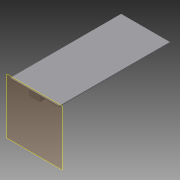
# Autodesk Inventor part: Flat Bearing
Saved by Autodesk Inventor 2014 (Build 180170000, 170)
## iProperties
Created: 2015-02-08
Part Number: Flat Bearing
Material: Generic
Document SubType Name: Modeling
Designer: Spooner
Density: 1 g/cm^3
Appearance: Default
Author: Spooner
Autodesk Inventor part; units mm, degrees
ref_plane "YZ Plane" through (0, 0, 0) normal (1, 0, 0) x (0, 1, 0)
ref_plane "XZ Plane" through (0, 0, 0) normal (0, 1, 0) x (-1, 0, 0)
ref_plane "XY Plane" through (0, 0, 0) normal (0, 0, 1) x (1, 0, 0)
ref_plane "Work Plane1" through (0, 0, 0) normal (0, 0, 1) x (1, 0, 0)
sketch "Sketch1" plane through (0, 0, 0) normal (0, 0, 1) x (1, 0, 0)
  circle A0 centre (0, 0) radius 2.413 projected
  line L0 (-4.7444, -6.5405) -> (4.7444, -6.5405) projected
  line L1 (4.7444, -6.5405) -> (10.16, -11.9561) projected
  line L2 (10.16, -11.9561) -> (10.16, -16.002) projected
  line L3 (10.16, -16.002) -> (6.985, -16.002) projected
  line L4 (6.985, -16.002) -> (6.985, -15.24) projected
  line L5 (6.985, -15.24) -> (4.445, -15.24) projected
  line L6 (4.445, -15.24) -> (4.445, -19.05) projected
  line L7 (4.445, -19.05) -> (19.05, -19.05) projected
  line L8 (19.05, -19.05) -> (19.05, -4.445) projected
  line L9 (19.05, -4.445) -> (15.24, -4.445) projected
  line L10 (15.24, -4.445) -> (15.24, -6.985) projected
  line L11 (15.24, -6.985) -> (16.002, -6.985) projected
  line L12 (16.002, -6.985) -> (16.002, -10.16) projected
  line L13 (16.002, -10.16) -> (11.9561, -10.16) projected
  line L14 (11.9561, -10.16) -> (6.5405, -4.7444) projected
  line L15 (6.5405, -4.7444) -> (6.5405, 4.7444) projected
  line L16 (6.5405, 4.7444) -> (11.9561, 10.16) projected
  line L17 (11.9561, 10.16) -> (16.002, 10.16) projected
  line L18 (16.002, 10.16) -> (16.002, 6.985) projected
  line L19 (16.002, 6.985) -> (15.24, 6.985) projected
  line L20 (15.24, 6.985) -> (15.24, 4.445) projected
  line L21 (15.24, 4.445) -> (19.05, 4.445) projected
  line L22 (19.05, 4.445) -> (19.05, 19.05) projected
  line L23 (19.05, 19.05) -> (4.445, 19.05) projected
  line L24 (4.445, 19.05) -> (4.445, 15.24) projected
  line L25 (4.445, 15.24) -> (6.985, 15.24) projected
  line L26 (6.985, 15.24) -> (6.985, 16.002) projected
  line L27 (6.985, 16.002) -> (10.16, 16.002) projected
  line L28 (10.16, 16.002) -> (10.16, 11.9561) projected
  line L29 (10.16, 11.9561) -> (4.7444, 6.5405) projected
  line L30 (4.7444, 6.5405) -> (-4.7444, 6.5405) projected
  line L31 (-4.7444, 6.5405) -> (-10.16, 11.9561) projected
  line L32 (-10.16, 11.9561) -> (-10.16, 16.002) projected
  line L33 (-10.16, 16.002) -> (-6.985, 16.002) projected
  line L34 (-6.985, 16.002) -> (-6.985, 15.24) projected
  line L35 (-6.985, 15.24) -> (-4.445, 15.24) projected
  line L36 (-4.445, 15.24) -> (-4.445, 19.05) projected
  line L37 (-4.445, 19.05) -> (-19.05, 19.05) projected
  line L38 (-19.05, 19.05) -> (-19.05, 4.445) projected
  line L39 (-19.05, 4.445) -> (-15.24, 4.445) projected
  line L40 (-15.24, 4.445) -> (-15.24, 6.985) projected
  line L41 (-15.24, 6.985) -> (-16.002, 6.985) projected
  line L42 (-16.002, 6.985) -> (-16.002, 10.16) projected
  line L43 (-16.002, 10.16) -> (-11.9561, 10.16) projected
  line L44 (-11.9561, 10.16) -> (-6.5405, 4.7444) projected
  line L45 (-6.5405, 4.7444) -> (-6.5405, -4.7444) projected
  line L46 (-6.5405, -4.7444) -> (-11.9561, -10.16) projected
  line L47 (-11.9561, -10.16) -> (-16.002, -10.16) projected
  line L48 (-16.002, -10.16) -> (-16.002, -6.985) projected
  line L49 (-16.002, -6.985) -> (-15.24, -6.985) projected
  line L50 (-15.24, -6.985) -> (-15.24, -4.445) projected
  line L51 (-15.24, -4.445) -> (-19.05, -4.445) projected
  line L52 (-19.05, -4.445) -> (-19.05, -19.05) projected
  line L53 (-19.05, -19.05) -> (-4.445, -19.05) projected
  line L54 (-4.445, -19.05) -> (-4.445, -15.24) projected
  line L55 (-4.445, -15.24) -> (-6.985, -15.24) projected
  line L56 (-6.985, -15.24) -> (-6.985, -16.002) projected
  line L57 (-6.985, -16.002) -> (-10.16, -16.002) projected
  line L58 (-10.16, -16.002) -> (-10.16, -11.9561) projected
  line L59 (-10.16, -11.9561) -> (-4.7444, -6.5405) projected
  line L60 (-18.415, 19.0754) -> (-4.191, 19.0754)
  line L61 (-4.191, 19.0754) -> (-4.191, 15.2146)
  line L62 (-4.191, 15.2146) -> (4.191, 15.2146)
  line L63 (4.191, 15.2146) -> (4.191, 19.0754)
  line L64 (4.191, 19.0754) -> (18.415, 19.0754)
  line L65 (18.415, 19.0754) -> (18.415, 19.6754)
  line L66 (18.415, 19.6754) -> (-18.415, 19.6754)
  line L67 (-18.415, 19.6754) -> (-18.415, 19.0754)
  dimension "d0" = 0.635
  dimension "d1" = 0.635
  dimension "d2" = 0.0254
  dimension "d3" = 0.6
  dimension "d4" = 0.254
  dimension "d5" = 0.254
  dimension "d6" = 0.0254
  constraints: 16 end point, 5 parallel, 2 perpendicular, 1 collinear, 1 horizontal alignment
  measures "d0" horizontal distance of L60.start L37.end
  measures "d1" horizontal distance of L22.end L64.end
  measures "d2" distance between parallel lines of L37 L60
  measures "d3" distance between parallel lines of L60 L66
  measures "d4" distance between parallel lines of L36 L61
  measures "d5" distance between parallel lines of L24 L63
  measures "d6" distance between parallel lines of L35 L62
extrude "Extrusion1" add sketch "Sketch1" against normal blind 83.82 contours L67 L66 L65 L64 L63 L62 L61 L60
equation "\"d1\" = d0"
equation "\"d5\" = d4"
equation "\"d6\" = d2"
body "Solid1"
